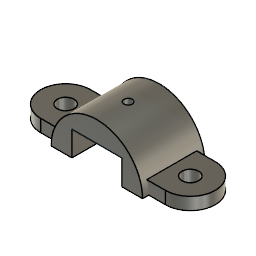
6- CREATE A SOLID 3D MODEL FROM ORTHOGRAPHIC PROJECTION (Autodesk Fusion 360 design; units mm, degrees)
part number: 2025-10-03-13-21-34-888
Autodesk Fusion 360 part; units mm, degrees
sketch "Sketch1" plane through (0, 0, 0) normal (0, 1, 0) x (1, 0, 0)
  line L0 (-60, 0) -> (-60, -60)
  line L1 (-60, -60) -> (60, -60)
  line L2 (60, -60) -> (60, 0)
  line L3 (60, 60) -> (-60, -60) construction
  line L4 (-60, 60) -> (60, -60) construction
  arc A0 (-110, 0) -> (110, 0) centre (0, 0) ccw
  line L5 (-110, 0) -> (0, 0)
  line L6 (60, 0) -> (110, 0)
  dimension "d1" = 220
  dimension "d2" = 120
  dimension "d3" = 120
  constraint coincident A0.centre L5.end
  constraint parallel L0 L2
  constraint coincident L3 A0.centre
  constraint coincident L4 A0.centre
  constraint perpendicular L2 L5
  constraint coincident L0.start L5
  constraint coincident L2.end L5
  constraint collinear L5 L6
  measures "d1" diameter of A0
  measures "d2" distance of L0.end L1.end
  measures "d3" distance of L4.start L0.end
extrude "Extrude1" add sketch "Sketch1" along normal mid plane 150 makes body 1
sketch "Sketch2" plane through (0, 0, 60) normal (0, 0, -1) x (1, 0, 0)
  line L0 (-60, 75) -> (-60, -75)
  line L1 (-60, -75) -> (60, -75)
  line L2 (60, -75) -> (60, 75)
  line L3 (60, 75) -> (-60, 75)
  circle A0 centre (0, 0) radius 10
  dimension "d6" = 20
  constraint coincident A0.centre origin
  measures "d6" diameter of A0
extrude "Extrude2" cut sketch "Sketch2" against normal blind 60 contours A0 bodies 1
sketch "Sketch3" plane through (0, 0, 60) normal (0, 0, -1) x (1, 0, 0)
  circle A0 centre (0, 0) radius 10
  line L0 (-60, 75) -> (-60, -75)
  line L1 (-60, -75) -> (60, -75)
  line L2 (60, -75) -> (60, 75)
  line L3 (60, 75) -> (-60, 75)
sketch "Sketch4" plane through (0, 0, 60) normal (0, 0, -1) x (1, 0, 0)
sketch "Sketch5" plane through (0, 0, 0) normal (0, 0, 1) x (1, 0, 0)
sketch "Sketch6" plane through (0, 0, 0) normal (0, 0, 1) x (1, 0, 0)
  line L0 (-210, 0) -> (223.8586, 0)
  line L1 (0, 130) -> (0, -130)
  circle A0 centre (150, 0) radius 20
  line L2 (150, 60) -> (105, 60)
  line L3 (150, -60) -> (105, -60)
  arc A1 (150, -60) -> (150, 60) centre (150, 0) ccw
  line L4 (105, 60) -> (105, -60)
  dimension "d10" = 40
  dimension "d11" = 150
  constraint horizontal L0
  constraint vertical L1
  constraint coincident L0 A0.centre
  constraint concentric A0 A1
  constraint tangent L2 A1
  constraint horizontal L2
  constraint tangent L3 A1
  constraint horizontal L3
  constraint perpendicular L3 L4
  measures "d10" diameter of A0
  measures "d11" distance of A0.centre origin
extrude "Extrude3" add sketch "Sketch6" along normal blind 30 separate body contours L0 A0 L2 A1 L4 | L0 A0 L3 A1 L4 makes body 2
sketch "Sketch7" plane through (0, 0, 0) normal (0, 0, 1) x (1, 0, 0)
  circle A0 centre (-150, 0) radius 20
  line L0 (-150, 60) -> (-105, 60)
  line L1 (-150, -60) -> (-105, -60)
  line L2 (-105, -60) -> (-105, 60)
  arc A1 (-150, 60) -> (-150, -60) centre (-150, 0) ccw
  dimension "d14" = 120
  dimension "d15" = 40
  dimension "d16" = 150
  constraint concentric A0 A1
  constraint tangent L0 A1
  constraint horizontal L0
  constraint tangent L1 A1
  constraint horizontal L1
  constraint perpendicular L0 L2
  measures "d14" diameter of A1
  measures "d15" diameter of A0
  measures "d16" distance of A0.centre origin
extrude "Extrude4" add sketch "Sketch7" along normal blind 30 separate body makes body 3
component "6- CREATE A SOLID 3D MODEL FROM ORTHOGRAPHIC PROJECTION" placed x (1, 0, 0) y (0, 1, 0) z (0, 0, 1) at (0, 0, 0)
